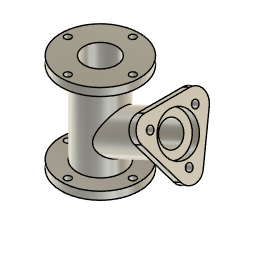
Flange (Autodesk Fusion 360 design; units mm, degrees)
part number: 2025-07-07-18-10-03-370
Autodesk Fusion 360 part; units mm, degrees
sketch "rev 1" plane through (0, 0, 0) normal (0, 1, 0) x (1, 0, 0)
  line L0 (0, 0) -> (60, 0)
  line L1 (60, 0) -> (60, -12)
  line L2 (60, -12) -> (35, -12)
  line L3 (35, -12) -> (35, -138)
  line L4 (35, -138) -> (60, -138)
  line L5 (60, -138) -> (60, -150)
  line L6 (60, -150) -> (0, -150)
  line L7 (0, -150) -> (0, 0)
  dimension "d18" = 60
  dimension "d19" = 12
  dimension "d20" = 126
  dimension "d21" = 12
  dimension "d22" = 35
  constraint coincident L0.start L7.end
  constraint horizontal L0
  constraint perpendicular L0 L1
  constraint perpendicular L1 L2
  constraint perpendicular L0 L3
  constraint perpendicular L1 L4
  constraint perpendicular L4 L5
  constraint perpendicular L5 L6
  constraint perpendicular L0 L7
  measures "d18" distance of L0.start L0.end
  measures "d19" distance of L0.end L1.end
  measures "d20" distance of L2.end L3.end
  measures "d21" distance of L4.end L5.end
  measures "d22" distance of L3 L7
revolve "Revolve1" add sketch "rev 1" angle 360 about axis through (0, 0, 150) along (0, 0, -1)
sketch "top cly" plane through (0, 0, 150) normal (0, 0, 1) x (-1, 0, 0)
  circle A0 centre (0, 0) radius 60
  circle A1 centre (0, 0) radius 25
  dimension "d24" = 50
  constraint concentric A0 A1
  measures "d24" diameter of A1
extrude "Extrude3" cut sketch "top cly" against normal through all contours A1
sketch "ext hole" plane through (0, 0, 150) normal (0, 0, 1) x (-1, 0, 0)
  circle A0 centre (0, 0) radius 25
  circle A1 centre (0, 0) radius 60
  circle A2 centre (0, 0) radius 50 construction
  circle A3 centre (0, -50) radius 5
  dimension "d26" = 100
  dimension "d27" = 10
  constraint concentric A0 A2
  constraint coincident A2 A3.centre
  measures "d26" diameter of A2
  measures "d27" diameter of A3
extrude "Extrude4" cut sketch "ext hole" against normal blind 170 contours A3
sketch "Sketch6" plane through (0, 0, 150) normal (0, 0, 1) x (-1, 0, 0)
  circle A0 centre (0, -50) radius 5
  circle A1 centre (0, 0) radius 25
  circle A2 centre (0, 0) radius 60
pattern_circular "C-Pattern2" count 4 over 360 about axis through (0, 0, 12) along (0, 0, 1) of "Extrude4"
sketch "Sketch18" plane through (0, 0, 0) normal (1, 0, 0) x (0, 1, 0)
sketch "Sketch20" plane through (0, 0, 0) normal (0, 1, 0) x (1, 0, 0)
  line L0 (0, -50) -> (108.7569, -100.7142) construction
  line L1 (0, -50) -> (180, -50) construction
  dimension "d63" = 25
  dimension "d64" = 120
  dimension "d65" = 50
  constraint horizontal L1
  measures "d63" angle of L0 L1
  measures "d64" distance of L0.start L0.end
  measures "d65" vertical distance of origin L0.start
ref_plane "WorkPlane7" through (108.7569, 0, 100.7142) normal (0.906308, 0, 0.422618) x (0, 1, 0)
sketch "Sketch21" plane through (108.7569, 0, 100.7142) normal (0.906308, 0, 0.422618) x (0, 1, 0)
  circle A0 centre (0, 0) radius 30
  dimension "d67" = 60
  constraint coincident A0.centre origin
  measures "d67" diameter of A0
extrude "Extrude10" add sketch "Sketch21" along normal up to surface and the other way blind -12 end surface at (34.9565, 1.7446, 54)
sketch "Sketch22" plane through (108.7569, 0, 100.7142) normal (0.906308, 0, 0.422618) x (0, 1, 0)
  circle A0 centre (0, 0) radius 18
  dimension "d70" = 36
  constraint coincident A0.centre origin
  measures "d70" diameter of A0
extrude "Extrude11" cut sketch "Sketch22" along normal blind -100 and the other way blind -70
sketch "Sketch23" plane through (108.7569, 0, 100.7142) normal (0.906308, 0, 0.422618) x (0, 1, 0)
  circle A0 centre (0, 0) radius 40 construction
  dimension "d73" = 80
  measures "d73" diameter of A0
sketch "Sketch24" plane through (108.7569, 0, 100.7142) normal (0.906308, 0, 0.422618) x (0, 1, 0)
  line L0 (-51.9615, 10) -> (-17.3205, -50)
  line L1 (17.3205, -50) -> (51.9615, 10)
  line L2 (34.641, 40) -> (-34.641, 40)
  arc A0 (-34.641, 40) -> (-51.9615, 10) centre (-34.641, 20) ccw
  arc A1 (51.9615, 10) -> (34.641, 40) centre (34.641, 20) ccw
  arc A2 (-17.3205, -50) -> (17.3205, -50) centre (0, -40) ccw
  circle A3 centre (-34.641, 20) radius 5.4
  line L3 (0, 0) -> (0, -76.0713)
  circle A4 centre (34.641, 20) radius 5.4
  circle A5 centre (0, -40) radius 5.4
  dimension "d74" = 20
  dimension "d75" = 10.8
  dimension "d76" = 10.8
  constraint coincident L3.start origin
  constraint tangent L0 A0
  constraint tangent L2 A0
  constraint tangent L2 A1
  constraint tangent L1 A1
  constraint equal A0 A1
  constraint tangent L1 A2
  constraint tangent L0 A2
  constraint equal A0 A2
  constraint concentric A0 A3
  constraint symmetric A3 L3 A4
  constraint concentric A2 A5
  measures "d74" radius of A0
  measures "d75" diameter of A3
  measures "d76" diameter of A5
extrude "Extrude12" add sketch "Sketch24" along normal blind 12
sketch "Sketch25" plane through (138.7837, 0, 64.7159) normal (0.906308, 0, 0.422618) x (0, 1, 0)
  circle A0 centre (34.641, 65.3154) radius 5.4
  circle A1 centre (0, 5.3154) radius 5.4
  circle A2 centre (-34.641, 65.3154) radius 5.4
  arc A3 (-17.3205, -4.6846) -> (17.3205, -4.6846) centre (0, 5.3154) ccw
  line L0 (17.3205, -4.6846) -> (51.9615, 55.3154)
  arc A4 (51.9615, 55.3154) -> (34.641, 85.3154) centre (34.641, 65.3154) ccw
  line L1 (34.641, 85.3154) -> (-34.641, 85.3154)
  arc A5 (-34.641, 85.3154) -> (-51.9615, 55.3154) centre (-34.641, 65.3154) ccw
  line L2 (-51.9615, 55.3154) -> (-17.3205, -4.6846)
  circle A6 centre (0, 45.3154) radius 30
  circle A7 centre (0, 45.3154) radius 18
  circle A8 centre (0, 45.3154) radius 30
  circle A9 centre (0, 45.3154) radius 18
  constraint concentric A7 A8
  constraint concentric A7 A9
extrude "Extrude13" cut sketch "Sketch25" against normal blind 12 contours A6 A8
extrude "Extrude14" cut 1 faces at (117.8636, 3, 109.5793) along direction (-0.906308, 0, -0.422618) blind 120
sketch "Sketch26" plane through (138.7837, 0, 64.7159) normal (0.906308, 0, 0.422618) x (0, 1, 0)
  circle A0 centre (0, 45) radius 18
  dimension "d87" = 36
  measures "d87" diameter of A0
